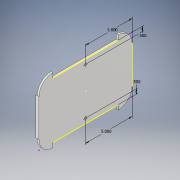
# Autodesk Inventor part: Frame 2.0
Saved by Autodesk Inventor 2018.2 (Build 222227000, 227)
## iProperties
Created: 2018-02-01
Part Number: Frame 2.0
Material: ABS Plastic
Document SubType Name: Modeling
Designer: MIABo
Density: 1.06 g/cm^3
Appearance: Smooth - White
Mass: 511.869 g
Surface Area: 864.604 cm^2
Volume: 482.895 cm^3
Author: MIABo
Autodesk Inventor part; units mm, degrees
ref_plane "YZ Plane" through (0, 0, 0) normal (1, 0, 0) x (0, 1, 0)
ref_plane "XZ Plane" through (0, 0, 0) normal (0, 1, 0) x (-1, 0, 0)
ref_plane "XY Plane" through (0, 0, 0) normal (0, 0, 1) x (1, 0, 0)
sketch "Sketch1" plane through (0, 0, 0) normal (1, 0, 0) x (0, 1, 0)
  line L0 (-76.2, 88.9) -> (-76.2, 88.9)
  line L1 (-50.8, 127) -> (50.8, 127)
  line L2 (50.8, -127) -> (-50.8, -127)
  line L3 (-76.2, -88.9) -> (-76.2, 88.9)
  arc A0 (88.9, 88.9) -> (50.8, 127) centre (50.8, 88.9) ccw
  line L4 (76.2, 88.9) -> (88.9, 88.9)
  arc A1 (-50.8, 127) -> (-88.9, 88.9) centre (-50.8, 88.9) ccw
  line L5 (-50.8, 88.9) -> (-88.9, 88.9)
  arc A2 (50.8, -127) -> (88.9, -88.9) centre (50.8, -88.9) ccw
  line L6 (76.2, -88.9) -> (88.9, -88.9)
  line L7 (76.2, 88.9) -> (76.2, -88.9)
  arc A3 (-88.9, -88.9) -> (-50.8, -127) centre (-50.8, -88.9) ccw
  line L8 (-76.2, -88.9) -> (-88.9, -88.9)
  point P0 (0, 0)
  point P1 (-76.2, 117.2981)
  point P2 (-76.2, -117.2981)
  dimension "d62" = 254
  dimension "d64" = 76.2
  dimension "d65" = 127
  dimension "d66" = 76.2
  dimension "d72" = 76.2
  dimension "d73" = 25.4
  dimension "d74" = 76.2
  dimension "d76" = 25.4
  dimension "d77" = 76.2
  dimension "d78" = 25.4
  constraints: 18 end point, 10 point on circle, 4 centre point, 4 horizontal, 4 tangent, 2 parallel, 2 perpendicular, 1 point on line
  measures "d62" distance between parallel lines of L2 L1
  measures "d64" distance from line of L3 point (0, 0)
  measures "d65" distance from line of L1 point (0, 0)
  measures "d66" diameter of A0
  measures "d72" diameter of A1
  measures "d73" distance from line of L3 L5.start
  measures "d74" diameter of A2
  measures "d76" distance from line of A2.centre L7
  measures "d77" diameter of A3
  measures "d78" distance from line of L3 A3.centre
extrude "Extrusion1" add sketch "Sketch1" along normal blind 5.08
sketch "Sketch3" plane through (5.08, 0, 0) normal (1, 0, 0) x (0, 0, -1)
  line L0 (88.9, 76.2) -> (-88.9, 76.2) projected
  line L1 (127, -50.8) -> (127, 50.8) projected
  line L2 (-88.9, -76.2) -> (88.9, -76.2) projected
  point P0 (0, 0)
  point P1 (0, -63.5)
  point P2 (0, 63.5)
  point P3 (0, 63.5)
  point P4 (127, 76.2)
  point P5 (127, -76.2)
  point P6 (-127, -76.2)
  dimension "d68" = 12.7
  dimension "d69" = 127
  dimension "d70" = 127
  dimension "d71" = 12.7
  constraints: 1 coincident
  measures "d68" distance from line of L0 point (0, 63.5)
  measures "d69" distance from line of L1 point (0, -63.5)
  measures "d70" distance from line of L1 point (0, 63.5)
  measures "d71" distance from line of L2 point (0, -63.5)
hole "Hole2" at (5.08, -63.5, 0) direction (-1, 0, 0) diameter 6.35 end through all
hole "Hole3" at (5.08, 63.5, 0) direction (-1, 0, 0) diameter 6.35 end through all
sketch "Sketch4" plane through (5.08, 0, 0) normal (1, 0, 0) x (0, 0, -1)
  line L0 (-127, 50.8) -> (-127, -50.8) projected
  line L1 (-127, 50.8) -> (127, 50.8)
  line L2 (127, 50.8) -> (127, -50.8)
  line L3 (127, -50.8) -> (-127, -50.8)
  line L4 (-127, -50.8) -> (-127, 50.8)
  point P0 (0, 0)
  point P1 (-88.9, 88.9)
  dimension "d79" = 101.6
  dimension "d80" = 38.1
  constraints: 8 end point, 2 parallel, 1 horizontal, 1 perpendicular, 1 point on line
  measures "d79" distance of L1.end L2.end
  measures "d80" distance from line of L1 point (-88.9, 88.9)
extrude "Extrusion2" add sketch "Sketch4" against normal blind 8.255
body "Solid1"
